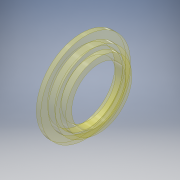
# Autodesk Inventor part: raccord rous libre
Saved by Autodesk Inventor 2018.1 (Build 221171000, 171)
## iProperties
Created: 2022-05-13
Part Number: raccord rous libre
Material: Generic
Document SubType Name: Modeling
Designer: Bureau
Density: 1 g/cm^3
Appearance: Default
Author: Bureau
Autodesk Inventor part; units mm, degrees
ref_plane "YZ Plane" through (0, 0, 0) normal (1, 0, 0) x (0, 1, 0)
ref_plane "XZ Plane" through (0, 0, 0) normal (0, 1, 0) x (-1, 0, 0)
ref_plane "XY Plane" through (0, 0, 0) normal (0, 0, 1) x (1, 0, 0)
sketch "Sketch1" plane through (0, 0, 0) normal (0, 0, 1) x (1, 0, 0)
  line L0 (0, 0) -> (10, 0)
  line L1 (0, 23) -> (5, 23)
  line L2 (5, 23) -> (5, 18.5)
  line L3 (12, 18.5) -> (12, 22.5)
  line L4 (12, 22.5) -> (9.5, 22.5)
  line L5 (0, 30.5) -> (0, 23)
  line L6 (5, 18.5) -> (12, 18.5)
  line L7 (0, 30.5) -> (3, 30.5)
  line L8 (3, 30.5) -> (3, 25.5)
  line L9 (3, 25.5) -> (8, 25.5)
  line L10 (8, 25.5) -> (8, 22.5)
  line L11 (8, 22.5) -> (9.5, 22.5)
  dimension "d0" = 10
  dimension "d1" = 23
  dimension "d2" = 5
  dimension "d4" = 7
  dimension "d9" = 4.5
  dimension "d10" = 18.5
  dimension "d11" = 3
  dimension "d12" = 5
  dimension "d13" = 5
  constraints: 24 end point, 5 perpendicular, 4 horizontal, 1 vertical
  measures "d0" distance of L0.start L0.end
  measures "d1" distance of L0.start L1.start
  measures "d2" distance of L1.start L1.end
  measures "d4" distance of L2.end L3.start
  measures "d9" distance of L1.end L2.end
  measures "d10" distance from line of L0 L2.end
  measures "d11" distance of L5.start L7.end
  measures "d12" distance of L7.end L8.end
  measures "d13" distance of L8.end L9.end
revolve "Revolution1" add sketch "Sketch1" angle 360 about axis through (0, 0, 0) along (1, 0, 0)
body "Solid1"
